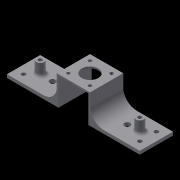
# Autodesk Inventor part: Base plate
Saved by Autodesk Inventor 2014 (Build 180170000, 170)
## iProperties
Created: 2014-11-03
Part Number: Base plate
Material: Generic
Document SubType Name: Modeling
Designer: Scott
Density: 1 g/cm^3
Appearance: Default
Author: Scott
Autodesk Inventor part; units mm, degrees
ref_plane "YZ Plane" through (0, 0, 0) normal (1, 0, 0) x (0, 1, 0)
ref_plane "XZ Plane" through (0, 0, 0) normal (0, 1, 0) x (-1, 0, 0)
ref_plane "XY Plane" through (0, 0, 0) normal (0, 0, 1) x (1, 0, 0)
sketch "Sketch1" plane through (0, 0, 0) normal (0, 1, 0) x (-1, 0, 0)
  line L0 (0, 0) -> (152.4, 0)
  line L1 (152.4, 0) -> (152.4, 50.8)
  line L2 (152.4, 50.8) -> (0, 50.8)
  line L3 (0, 50.8) -> (0, 0)
  dimension "d0" = 152.4
  dimension "d1" = 50.8
  constraints: 8 end point, 2 perpendicular, 1 horizontal, 1 parallel
  measures "d0" distance of L0.start L0.end
  measures "d1" distance of L0.end L1.end
extrude "Extrusion1" add sketch "Sketch1" along normal blind 5.08
sketch "Sketch2" plane through (0, 5.08, 0) normal (0, 1, 0) x (1, 0, 0)
  line L0 (0, 0) -> (-152.4, 0) projected
  line L1 (-152.4, -50.8) -> (0, -50.8) projected
  line L2 (-76.2, 0) -> (-76.2, -25.4)
  line L3 (-76.2, -25.4) -> (-59.69, -25.4)
  line L4 (-59.69, -25.4) -> (-59.69, -8.89)
  line L5 (-59.69, -8.89) -> (-53.34, -8.89)
  line L6 (-53.34, -8.89) -> (-53.34, -50.8)
  line L7 (-53.34, -8.89) -> (-53.34, 0)
  line L8 (-53.34, 0) -> (-50.8, 0)
  line L9 (-50.8, 0) -> (-50.8, -50.8)
  line L10 (-53.34, -50.8) -> (-50.8, -50.8)
  dimension "d4" = 16.51
  dimension "d5" = 16.51
  dimension "d6" = 6.35
  dimension "d7" = 2.54
  constraints: 18 end point, 6 perpendicular, 4 point on line, 2 collinear, 1 midpoint
  measures "d4" distance of L2.end L3.end
  measures "d5" distance of L3.end L4.end
  measures "d6" distance of L4.end L5.end
  measures "d7" distance of L7.end L8.end
extrude "Extrusion2" add sketch "Sketch2" along normal blind 36.83 contours L9 L1 L6 L7 L0
sketch "Sketch3" plane through (0, 5.08, 0) normal (0, 1, 0) x (1, 0, 0)
  line L0 (-53.34, 0) -> (-152.4, 0) projected
  line L1 (-152.4, -50.8) -> (-53.34, -50.8) projected
  line L2 (-152.4, 0) -> (-76.2, 0)
  line L3 (-76.2, 0) -> (-76.2, -25.4)
  line L4 (-76.2, -25.4) -> (-92.71, -25.4)
  line L5 (-92.71, -25.4) -> (-99.06, -25.4)
  line L6 (-99.06, -25.4) -> (-99.06, 0)
  line L7 (-99.06, 0) -> (-101.6, 0)
  line L8 (-101.6, 0) -> (-101.6, -50.8)
  line L9 (-101.6, -50.8) -> (-99.06, -50.8)
  line L10 (-99.06, -25.4) -> (-99.06, -50.8)
  point P0 (0, 0)
  dimension "d10" = 76.2
  dimension "d11" = 16.51
  dimension "d12" = 6.35
  dimension "d13" = 2.54
  constraints: 18 end point, 6 point on line, 4 perpendicular, 1 parallel
  measures "d10" distance of L0.end L2.end
  measures "d11" distance of L3.end L4.end
  measures "d12" distance of L4.end L5.end
  measures "d13" distance of L6.end L7.end
extrude "Extrusion3" add sketch "Sketch3" along normal blind 36.83 contours L6 L10 L1 L8 L0
sketch "Sketch4" plane through (0, 41.91, 0) normal (0, 1, 0) x (1, 0, 0)
  line L0 (-101.6, 0) -> (-101.6, -50.8) projected
  line L1 (-101.6, 0) -> (-50.8, 0)
  line L2 (-50.8, 0) -> (-50.8, -50.8)
  line L3 (-50.8, -50.8) -> (-101.6, -50.8)
  point P0 (0, 0)
  dimension "d16" = 50.8
  constraints: 6 end point, 2 perpendicular, 1 parallel
  measures "d16" distance of L0.start L1.end
extrude "Extrusion4" add sketch "Sketch4" along normal blind 2.54
sketch "Sketch5" plane through (0, 5.08, 0) normal (0, 1, 0) x (1, 0, 0)
  line L0 (-99.06, 0) -> (-99.06, -50.8) projected
  line L1 (-99.06, -50.8) -> (-53.34, -50.8) projected
  line L2 (-53.34, -50.8) -> (-53.34, 0) projected
  line L3 (-53.34, 0) -> (-99.06, 0) projected
  point P0 (0, 0)
extrude "Extrusion5" cut sketch "Sketch5" against normal blind 13.6525
sketch "Sketch6" plane through (0, 44.45, 0) normal (0, 1, 0) x (1, 0, 0)
  line L0 (-50.8, 0) -> (-101.6, 0) projected
  line L1 (-101.6, 0) -> (-101.6, -50.8) projected
  line L2 (-76.2, 0) -> (-76.2, -25.4)
  circle A0 centre (-76.2, -25.4) radius 12.7
  line L3 (-76.2, -25.4) -> (-59.69, -25.4)
  line L4 (-59.69, -25.4) -> (-59.69, -8.89)
  circle A1 centre (-59.69, -8.89) radius 2.54
  line L5 (-59.69, -25.4) -> (-59.69, -41.91)
  circle A2 centre (-59.69, -41.91) radius 2.54
  line L6 (-76.2, -25.4) -> (-92.71, -25.4)
  line L7 (-92.71, -25.4) -> (-92.71, -8.89)
  circle A3 centre (-92.71, -8.89) radius 2.54
  line L8 (-92.71, -25.4) -> (-92.71, -41.91)
  circle A4 centre (-92.71, -41.91) radius 2.54
  point P0 (0, 0)
  dimension "d21" = 25.4
  dimension "d22" = 16.51
  dimension "d23" = 16.51
  dimension "d24" = 5.08
  dimension "d25" = 16.51
  dimension "d26" = 5.08
  dimension "d27" = 16.51
  dimension "d28" = 16.51
  dimension "d29" = 5.08
  dimension "d30" = 16.51
  dimension "d31" = 5.08
  constraints: 14 end point, 5 centre point, 5 coincident, 4 perpendicular, 2 collinear, 1 midpoint, 1 parallel
  measures "d21" diameter of A0
  measures "d22" distance of L3.start L3.end
  measures "d23" distance of L3.end L4.end
  measures "d24" diameter of A1
  measures "d25" distance of L3.end L5.end
  measures "d26" diameter of A2
  measures "d27" distance of L3.start L6.end
  measures "d28" distance of L6.end L7.end
  measures "d29" diameter of A3
  measures "d30" distance of L6.end L8.end
  measures "d31" diameter of A4
extrude "Extrusion6" cut sketch "Sketch6" against normal blind 13.6525
sketch "Sketch7" plane through (0, 5.08, 0) normal (0, 1, 0) x (1, 0, 0)
  line L0 (0, -50.8) -> (0, 0) projected
  line L1 (0, 0) -> (-50.8, 0) projected
  line L2 (0, 0) -> (25.4, 0)
  line L3 (25.4, 0) -> (25.4, -50.8)
  line L4 (25.4, -50.8) -> (0, -50.8)
  dimension "d34" = 25.4
  constraints: 6 end point, 1 collinear, 1 parallel, 1 perpendicular
  measures "d34" distance of L0.end L2.end
extrude "Extrusion7" add sketch "Sketch7" against normal blind 5.08
sketch "Sketch8" plane through (-152.4, 0, 0) normal (-1, 0, 0) x (0, 0, 1)
  line L0 (0, 0) -> (50.8, 0) projected
  line L1 (50.8, 0) -> (50.8, 5.08) projected
  line L2 (0, 5.08) -> (50.8, 5.08) projected
  line L3 (0, 0) -> (0, 5.08) projected
extrude "Extrusion8" add sketch "Sketch8" along normal blind 25.4
sketch "Sketch9" plane through (0, 5.08, 0) normal (0, 1, 0) x (1, 0, 0)
  line L0 (-101.6, 0) -> (-177.8, 0) projected
  line L1 (-101.6, 0) -> (-152.4, 0)
  line L2 (-152.4, 0) -> (-152.4, -25.4)
  circle A0 centre (-152.4, -25.4) radius 6
  circle A1 centre (-152.4, -25.4) radius 3
  point P0 (0, 0)
  dimension "d39" = 50.8
  dimension "d40" = 12
  dimension "d41" = 6
  constraints: 4 end point, 2 centre point, 2 coincident, 1 perpendicular, 1 point on line
  measures "d39" distance of L0.start L1.end
  measures "d40" diameter of A0
  measures "d41" diameter of A1
extrude "Extrusion9" add sketch "Sketch9" along normal blind 19.05
sketch "Sketch10" plane through (0, 5.08, 0) normal (0, 1, 0) x (1, 0, 0)
  line L0 (25.4, 0) -> (-50.8, 0) projected
  line L1 (-50.8, 0) -> (0, 0)
  line L2 (0, 0) -> (0, -25.4)
  line L3 (0, -25.4) -> (0, 0)
  circle A0 centre (0, -25.4) radius 3
  circle A1 centre (0, -25.4) radius 6
  dimension "d44" = 50.8
  dimension "d45" = 6
  dimension "d46" = 12
  constraints: 6 end point, 2 centre point, 2 coincident, 2 collinear, 1 perpendicular
  measures "d44" distance of L0.end L1.end
  measures "d45" diameter of A0
  measures "d46" diameter of A1
extrude "Extrusion10" add sketch "Sketch10" along normal blind 19.05
fillet "Fillet1" radius 4.7625 2 edges at (-158.4, 5.08, 25.4) (-6, 5.08, 25.4)
fillet "Fillet2" radius 20.6375 2 edges at (-50.8, 5.08, 25.4) (-101.6, 5.08, 25.4)
sketch "Sketch11" plane through (0, 5.08, 0) normal (0, 1, 0) x (1, 0, 0)
  line L0 (-122.2375, 0) -> (-177.8, 0) projected
  line L1 (-122.2375, -50.8) -> (-177.8, -50.8) projected
  line L2 (-177.8, 0) -> (-165.1, 0)
  line L3 (-165.1, 0) -> (-165.1, -12.7)
  circle A0 centre (-165.1, -12.7) radius 3.175
  line L4 (-177.8, -50.8) -> (-165.1, -50.8)
  line L5 (-165.1, -50.8) -> (-165.1, -38.1)
  circle A1 centre (-165.1, -38.1) radius 3.175
  point P0 (0, 0)
  dimension "d51" = 12.7
  dimension "d52" = 12.7
  dimension "d53" = 6.35
  dimension "d54" = 12.7
  dimension "d55" = 12.7
  dimension "d56" = 6.35
  constraints: 8 end point, 2 centre point, 2 coincident, 2 perpendicular, 2 point on line
  measures "d51" distance of L0.end L2.end
  measures "d52" distance of L2.end L3.end
  measures "d53" diameter of A0
  measures "d54" distance of L1.end L4.end
  measures "d55" distance of L4.end L5.end
  measures "d56" diameter of A1
extrude "Extrusion11" cut sketch "Sketch11" against normal blind 19.05
sketch "Sketch12" plane through (0, 5.08, 0) normal (0, 1, 0) x (1, 0, 0)
  line L0 (-30.1625, -50.8) -> (25.4, -50.8) projected
  line L1 (25.4, 0) -> (-30.1625, 0) projected
  line L2 (25.4, 0) -> (12.7, 0)
  line L3 (12.7, 0) -> (12.7, -12.7)
  circle A0 centre (12.7, -12.7) radius 3.175
  line L4 (25.4, -50.8) -> (12.7, -50.8)
  line L5 (12.7, -50.8) -> (12.7, -38.1)
  circle A1 centre (12.7, -38.1) radius 3.175
  point P0 (0, 0)
  dimension "d59" = 12.7
  dimension "d60" = 12.7
  dimension "d61" = 6.35
  dimension "d62" = 12.7
  dimension "d63" = 12.7
  dimension "d64" = 6.35
  constraints: 8 end point, 2 centre point, 2 coincident, 2 perpendicular, 2 point on line
  measures "d59" distance of L1.start L2.end
  measures "d60" distance of L2.end L3.end
  measures "d61" diameter of A0
  measures "d62" distance of L0.end L4.end
  measures "d63" distance of L4.end L5.end
  measures "d64" diameter of A1
extrude "Extrusion12" cut sketch "Sketch12" against normal blind 19.05
sketch "Sketch13" plane through (0, 5.08, 0) normal (0, 1, 0) x (1, 0, 0)
  line L0 (-122.2375, 0) -> (-177.8, 0) projected
  line L1 (-177.8, 0) -> (-133.35, 0)
  line L2 (-133.35, 0) -> (-133.35, -25.4)
  circle A0 centre (-133.35, -25.4) radius 4.445
  point P0 (0, 0)
  dimension "d67" = 44.45
  dimension "d68" = 8.89
  constraints: 4 end point, 1 centre point, 1 coincident, 1 perpendicular, 1 point on line
  measures "d67" distance of L0.end L1.end
  measures "d68" diameter of A0
sketch "Sketch14" plane through (0, 5.08, 0) normal (0, 1, 0) x (1, 0, 0)
  line L0 (25.4, 0) -> (-30.1625, 0) projected
  line L1 (25.4, 0) -> (-19.05, 0)
  line L2 (-19.05, 0) -> (-19.05, -25.4)
  circle A0 centre (-19.05, -25.4) radius 4.445
  point P0 (0, 0)
  dimension "d69" = 44.45
  dimension "d70" = 8.89
  constraints: 4 end point, 1 centre point, 1 coincident, 1 perpendicular, 1 point on line
  measures "d69" distance of L0.start L1.end
  measures "d70" diameter of A0
extrude "Extrusion13" cut sketch "Sketch13" against normal blind 19.05
extrude "Extrusion14" cut sketch "Sketch14" against normal blind 19.05
body "Solid1"
